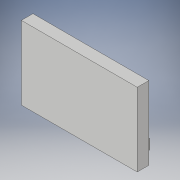
# Autodesk Inventor part: IMU
Saved by Autodesk Inventor 2017 (Build 210142000, 142)
## iProperties
Created: 2018-07-29
Part Number: IMU
Material: Generic
Document SubType Name: Modeling
Designer: Alexander Miller
Density: 1 g/cm^3
Appearance: Default
Author: Alexander Miller
Autodesk Inventor part; units mm, degrees
ref_plane "YZ Plane" through (0, 0, 0) normal (1, 0, 0) x (0, 1, 0)
ref_plane "XZ Plane" through (0, 0, 0) normal (0, 1, 0) x (-1, 0, 0)
ref_plane "XY Plane" through (0, 0, 0) normal (0, 0, 1) x (1, 0, 0)
sketch "Sketch1" plane through (0, 0, 0) normal (0, 0, 1) x (1, 0, 0)
  line L0 (-15, -9.5) -> (15, -9.5)
  line L1 (15, -9.5) -> (15, 9.5)
  line L2 (15, 9.5) -> (-15, 9.5)
  line L3 (-15, 9.5) -> (-15, -9.5)
  point P0 (0, 0)
  point P1 (0, 9.5)
  point P2 (15, 0)
  dimension "d0" = 30
  dimension "d1" = 19
  constraints: 8 end point, 2 midpoint, 2 parallel, 1 horizontal, 1 horizontal alignment, 1 perpendicular, 1 vertical alignment
  measures "d0" distance of L1.end L2.end
  measures "d1" distance of L0.end L1.end
extrude "Extrusion1" add sketch "Sketch1" along normal blind 3
sketch "Sketch2" plane through (0, 0, 0) normal (0, 0, -1) x (-1, 0, 0)
  line L0 (-12.7, -5.93) -> (12.7, -5.93)
  line L1 (12.7, -5.93) -> (12.7, -8.47)
  line L2 (12.7, -8.47) -> (-12.7, -8.47)
  line L3 (-12.7, -8.47) -> (-12.7, -5.93)
  line L4 (15, -9.5) -> (-15, -9.5) projected
  circle A0 centre (-11.46, -7.2) radius 0.5
  circle A1 centre (-8.92, -7.2) radius 0.5
  circle A2 centre (-6.38, -7.2) radius 0.5
  circle A3 centre (-3.84, -7.2) radius 0.5
  circle A4 centre (-1.3, -7.2) radius 0.5
  circle A5 centre (1.24, -7.2) radius 0.5
  circle A6 centre (3.78, -7.2) radius 0.5
  circle A7 centre (6.32, -7.2) radius 0.5
  circle A8 centre (8.86, -7.2) radius 0.5
  circle A9 centre (11.4, -7.2) radius 0.5
  line L5 (15, 9.5) -> (15, -9.5) projected
  point P0 (0, 0)
  point P1 (-12.7, -7.2)
  point P2 (0, -5.93)
  point P3 (12.7, -7.2)
  dimension "d4" = 2.3
  dimension "d5" = 2.54
  dimension "d6" = 25.4
  dimension "d7" = 3.6
  dimension "d8" = 2.54
  dimension "d9" = 2.54
  dimension "d10" = 2.54
  dimension "d11" = 2.54
  dimension "d12" = 2.54
  dimension "d13" = 2.54
  dimension "d14" = 2.54
  dimension "d15" = 2.54
  dimension "d16" = 2.54
  dimension "d17" = 1
  constraints: 10 centre point, 10 horizontal alignment, 9 equal radius, 8 end point, 3 midpoint, 2 parallel, 1 horizontal, 1 perpendicular, 1 vertical alignment
  measures "d4" distance from line of point (-12.7, -7.2) L4
  measures "d5" distance of L2.end L0.start
  measures "d6" distance of L0.start L0.end
  measures "d7" distance from line of A9.centre L5
  measures "d8" distance of A9.centre A8.centre
  measures "d9" distance of A8.centre A7.centre
  measures "d10" distance of A7.centre A6.centre
  measures "d11" distance of A6.centre A5.centre
  measures "d12" distance of A5.centre A4.centre
  measures "d13" distance of A4.centre A3.centre
  measures "d14" distance of A3.centre A2.centre
  measures "d15" distance of A2.centre A1.centre
  measures "d16" distance of A1.centre A0.centre
  measures "d17" diameter of A9
extrude "Extrusion2" add sketch "Sketch2" along normal blind 2.54
equation "\"d9\" = d8"
equation "\"d10\" = d8"
equation "\"d11\" = d8"
equation "\"d12\" = d8"
equation "\"d13\" = d8"
equation "\"d14\" = d8"
equation "\"d15\" = d8"
equation "\"d16\" = d8"
body "Solid1"
